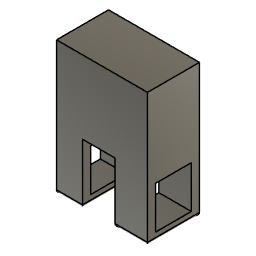
leg v11 v4 (Autodesk Fusion 360 design; units mm, degrees)
Autodesk Fusion 360 part; units mm, degrees
sketch "Sketch1" plane through (0, 0, 0) normal (0, 0, 1) x (1, 0, 0)
  line L0 (0, 0) -> (60, 0)
  line L1 (60, 0) -> (60, 20)
  line L2 (60, 20) -> (0, 20)
  line L3 (0, 20) -> (0, 0)
  dimension "d1" = 60
  dimension "d2" = 20
  constraint horizontal L0
  constraint vertical L1
  constraint horizontal L2
  constraint vertical L3
  constraint coincident L0.start L3.end
  measures "d1" distance of L0.start L0.end
  measures "d2" distance of L0.start L2.end
extrude "Extrude1" add sketch "Sketch1" along normal blind 40
sketch "Sketch2" plane through (0, 0, 0) normal (-1, 0, 0) x (0, -1, 0)
  line L0 (-20, 0) -> (0, 0)
  line L1 (0, 0) -> (0, 40)
  line L2 (0, 40) -> (-20, 40)
  line L3 (-20, 40) -> (-20, 0)
  line L4 (-15, 28) -> (-5, 28)
  line L5 (-5, 28) -> (-5, 16)
  line L6 (-5, 16) -> (-15, 16)
  line L7 (-15, 16) -> (-15, 28)
  dimension "d5" = 10
  dimension "d6" = 12
  dimension "d7" = 5
  constraint horizontal L4
  constraint vertical L5
  constraint horizontal L6
  constraint vertical L7
  measures "d5" distance of L4.start L4.end
  measures "d6" distance of L4.start L6.end
  measures "d7" distance of L3 L7
extrude "Extrude2" cut sketch "Sketch2" against normal blind 30 contours L4 L5 L6 L7
extrude "Extrude3" cut 1 faces at (20, 13.3333, 40) along direction (0, 0, -1) blind 2
extrude "Extrude4" cut 1 faces at (20, 13.3333, 0) along direction (0, 0, 1) blind 2
sketch "Sketch3" plane through (0, 20, 0) normal (0, 1, 0) x (-1, 0, 0)
  line L0 (-60, 2) -> (0, 2)
  line L1 (0, 2) -> (0, 38)
  line L2 (0, 38) -> (-60, 38)
  line L3 (-60, 38) -> (-60, 2)
  line L4 (-40, 33) -> (-20, 33)
  line L5 (-20, 33) -> (-20, -1)
  line L6 (-20, -1) -> (-40, -1)
  line L7 (-40, -1) -> (-40, 33)
  dimension "d14" = 20
  dimension "d15" = 34
  dimension "d16" = 20
  dimension "d17" = 5
  constraint horizontal L4
  constraint vertical L5
  constraint horizontal L6
  constraint vertical L7
  measures "d14" distance of L4.start L4.end
  measures "d15" distance of L4.start L6.end
  measures "d16" distance of L3 L7
  measures "d17" distance of L2 L4
extrude "Extrude5" cut 1 faces at (20, 13.3333, 2) along direction (0, 0, 1) blind 9
extrude "Extrude6" cut 1 faces at (20, 13.3333, 11) along direction (0, 0, 1) blind 1
extrude "Extrude7" cut sketch "Sketch3" against normal blind 20 contours L0 L4 L5 L7
extrude "Extrude8" cut sketch "Sketch2" against normal blind 80 contours L4 L5 L6 L7
extrude "Extrude9" cut 1 faces at (20, 13.3333, 38) along direction (0, 0, -1) blind 1
extrude "Extrude10" cut 1 faces at (60, 8.3333, 34) along direction (-1, 0, 0) blind 10
extrude "Extrude11" add 1 faces at (40, 1.6667, 24.3333) along direction (-1, 0, 0) blind 10
extrude "Extrude12" cut 1 faces at (50, 8.3333, 34) along direction (-1, 0, 0) blind 10
extrude "Extrude13" cut 1 faces at (6.6667, 20, 27.3333) along direction (0, -1, 0) blind 2
extrude "Extrude14" cut 1 faces at (6.6667, 0, 27.3333) along direction (0, 1, 0) blind 2
extrude "Extrude15" cut 1 faces at (36.6667, 12.6667, 12) along direction (0, 0, 1) blind 1
extrude "Extrude16" cut 1 faces at (13.3333, 7.3333, 12) along direction (0, 0, 1) blind 1
extrude "Extrude17" cut 1 faces at (36.6667, 12.6667, 13) along direction (0, 0, 1) blind 1
extrude "Extrude18" cut 1 faces at (13.3333, 7.3333, 13) along direction (0, 0, 1) blind 1
extrude "Extrude19" cut sketch "Sketch2" against normal blind 2
extrude "Extrude20" cut 1 faces at (14.6667, 7.3333, 37) along direction (0, 0, -1) blind 1
extrude "Extrude21" add 1 faces at (26.6667, 12.6667, 33) along direction (0, 0, -1) blind 1
extrude "Extrude22" cut 1 faces at (14.6667, 7.3333, 36) along direction (0, 0, -1) blind 1
fillet "Fillet1" radius 1 2 faces at (36.6667, 12.6667, 14) (14, 7.3333, 14)
sketch "Sketch4" plane through (2, 0, 0) normal (-1, 0, 0) x (0, -1, 0)
  line L0 (-5, 16) -> (-15, 16)
  line L1 (-15, 16) -> (-15, 28)
  line L2 (-15, 28) -> (-5, 28)
  line L3 (-5, 28) -> (-5, 16)
  line L4 (-18, 15) -> (-2, 15)
  line L5 (-2, 15) -> (-2, 35)
  line L6 (-2, 35) -> (-18, 35)
  line L7 (-18, 35) -> (-18, 15)
  line L8 (-15.5, 28.5) -> (-4.5, 28.5)
  line L9 (-4.5, 28.5) -> (-4.5, 15.5)
  line L10 (-4.5, 15.5) -> (-15.5, 15.5)
  line L11 (-15.5, 15.5) -> (-15.5, 28.5)
  dimension "d56" = 11
  dimension "d57" = 13
  dimension "d58" = 2.5
  dimension "d59" = 6.5
  constraint horizontal L8
  constraint vertical L9
  constraint horizontal L10
  constraint vertical L11
  measures "d56" distance of L8.start L8.end
  measures "d57" distance of L8.start L10.end
  measures "d58" distance of L7 L11
  measures "d59" distance of L6 L8
extrude "Extrude23" cut sketch "Sketch4" against normal blind 50 contours L8 L9 L10 L11
extrude "Extrude24" add 2 faces at (36.6667, 8.1667, 15.5) (14, 11.8333, 15.5) along direction (0, 0, 1) blind 1
extrude "Extrude25" cut 2 faces at (33.3333, 11.8333, 28.5) (14, 11.8333, 28.5) along direction (0, 0, 1) blind 1
extrude "Extrude26" cut 1 faces at (26.6667, 12.6667, 32) along direction (0, 0, 1) blind 0.5
extrude "Extrude27" add 1 faces at (14.6667, 7.3333, 35) along direction (0, 0, 1) blind 20
extrude "Extrude28" cut 1 faces at (2, 8.1667, 46.5) along direction (1, 0, 0) blind 10
extrude "Extrude29" cut 1 faces at (5.3333, 12.6667, 15) along direction (0, 0, -1) blind 15
